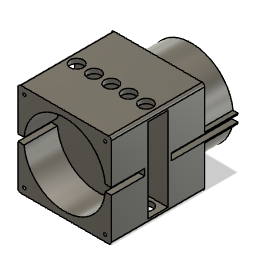
TWO MAG BODY 3x1 v13 (Autodesk Fusion 360 design; units mm, degrees)
Autodesk Fusion 360 part; units mm, degrees
sketch "Sketch3" plane through (0, 0, 0) normal (0, 0, 1) x (1, 0, 0)
  line L0 (44.45, 44.45) -> (-44.45, 44.45)
  line L1 (-44.45, 44.45) -> (-44.45, -44.45)
  line L2 (-44.45, -44.45) -> (44.45, -44.45)
  line L3 (44.45, -44.45) -> (44.45, 44.45)
  line L4 (44.45, 44.45) -> (-44.45, -44.45) construction
  line L5 (-44.45, 44.45) -> (44.45, -44.45) construction
  dimension "d6" = 88.9
  dimension "d7" = 88.9
  constraint perpendicular L0 L1
  constraint parallel L0 L2
  constraint parallel L1 L3
  constraint horizontal L0
  constraint coincident L4 origin
  constraint coincident L5 origin
  measures "d6" distance of L1.end L2.end
  measures "d7" distance of L0.end L1.end
extrude "Extrude2" add sketch "Sketch3" along normal mid plane 76.2
sketch "Sketch5" plane through (0, 0, 38.1) normal (0, 0, 1) x (1, 0, 0)
  line L0 (44.45, -44.45) -> (44.45, 44.45)
  line L1 (44.45, 44.45) -> (-44.45, 44.45)
  line L2 (-44.45, 44.45) -> (-44.45, -44.45)
  line L3 (-44.45, -44.45) -> (44.45, -44.45)
  circle A0 centre (0, 0) radius 38.735
  dimension "d14" = 77.47
  constraint coincident A0.centre origin
  measures "d14" diameter of A0
extrude "Extrude13" cut sketch "Sketch5" against normal blind 25.4 contours A0
sketch "Sketch10" plane through (44.45, 0, 0) normal (1, 0, 0) x (0, 0, -1)
  line L0 (38.1, 44.45) -> (-38.1, 44.45)
  line L1 (-38.1, 44.45) -> (-38.1, -44.45)
  line L2 (-38.1, -44.45) -> (38.1, -44.45)
  line L3 (38.1, -44.45) -> (38.1, 44.45)
  line L4 (9.525, 40.005) -> (-9.525, 40.005)
  line L5 (-9.525, 40.005) -> (-9.525, -40.005)
  line L6 (-9.525, -40.005) -> (9.525, -40.005)
  line L7 (9.525, -40.005) -> (9.525, 40.005)
  line L8 (9.525, 40.005) -> (-9.525, -40.005) construction
  line L9 (-9.525, 40.005) -> (9.525, -40.005) construction
  dimension "d42" = 80.01
  dimension "d43" = 19.05
  constraint perpendicular L4 L5
  constraint parallel L4 L6
  constraint parallel L5 L7
  constraint horizontal L4
  constraint coincident L8 origin
  constraint coincident L9 origin
  measures "d42" distance of L4.end L5.end
  measures "d43" distance of L5.end L6.end
extrude "Extrude9" cut sketch "Sketch10" against normal blind 88.9 contours L4 L5 L6 L7
sketch "Sketch6" plane through (0, 0, -38.1) normal (0, 0, -1) x (-1, 0, 0)
  line L0 (-44.45, 44.45) -> (-44.45, -44.45)
  line L1 (-44.45, -44.45) -> (44.45, -44.45)
  line L2 (44.45, -44.45) -> (44.45, 44.45)
  line L3 (44.45, 44.45) -> (-44.45, 44.45)
  circle A0 centre (0, 0) radius 38.735
  dimension "d17" = 77.47
  constraint coincident A0.centre origin
  measures "d17" diameter of A0
extrude "Extrude5" cut sketch "Sketch6" against normal blind 25.4 contours A0
sketch "Sketch7" plane through (44.45, 0, 0) normal (1, 0, 0) x (0, 0, -1)
  line L0 (38.1, 44.45) -> (-38.1, 44.45)
  line L1 (-38.1, 44.45) -> (-38.1, -44.45)
  line L2 (-38.1, -44.45) -> (38.1, -44.45)
  line L3 (38.1, -44.45) -> (38.1, 44.45)
  line L4 (-9.525, 40.005) -> (9.525, 40.005)
  line L5 (9.525, 40.005) -> (9.525, -40.005)
  line L6 (9.525, -40.005) -> (-9.525, -40.005)
  line L7 (-9.525, -40.005) -> (-9.525, 40.005)
  line L8 (-12.7, 3.175) -> (-12.7, -3.175)
  line L9 (-38.1, 3.175) -> (-38.1, -3.175)
  line L10 (12.7, -3.175) -> (12.7, 3.175)
  line L11 (38.1, -3.175) -> (38.1, 3.175)
  line L12 (12.7, 3.175) -> (38.1, 3.175)
  line L13 (38.1, -3.175) -> (12.7, -3.175)
  line L14 (-12.7, -3.175) -> (-38.1, -3.175)
  line L15 (-38.1, 3.175) -> (-12.7, 3.175)
  point P0 (-19.05, 0)
  constraint coincident L1 L9.start
  constraint coincident L1 L9.end
  constraint perpendicular L11 L12
  constraint perpendicular L10 L13
  constraint perpendicular L1 L14
  constraint perpendicular L8 L15
extrude "Extrude6" cut sketch "Sketch7" against normal blind 88.9 contours L3 L10 L11 L12 L13 | L1 L8 L9 L14 L15 | L4 L5 L6 L7
sketch "Sketch8" plane through (0, 0, 38.1) normal (0, 0, 1) x (1, 0, 0)
  line L0 (-44.45, -3.175) -> (-44.45, -44.45)
  line L1 (-44.45, -44.45) -> (44.45, -44.45)
  line L2 (44.45, -44.45) -> (44.45, -3.175)
  line L3 (-44.45, -44.45) -> (-44.45, -38.45) construction
  line L4 (-44.45, -38.45) -> (-38.45, -38.45) construction
  circle A0 centre (-38.45, -38.45) radius 1.4
  line L5 (0, 0) -> (0, -44.45) construction
  circle A1 centre (38.45, -38.45) radius 1.4
  circle A2 centre (38.45, 38.45) radius 1.4
  circle A3 centre (-38.45, 38.45) radius 1.4
  line L6 (44.45, -3.175) -> (38.6047, -3.175)
  arc A4 (-38.6047, -3.175) -> (38.6047, -3.175) centre (0, 0) ccw
  line L7 (-38.6047, -3.175) -> (-44.45, -3.175)
  dimension "d26" = 6
  dimension "d27" = 6
  dimension "d28" = 2.8
  dimension "d31" = 360
  constraint coincident L0.end L1.start
  constraint perpendicular L1 L3
  constraint perpendicular L3 L4
  constraint coincident L4.end A0.centre
  constraint midpoint L1 L5.end
  measures "d26" distance of L0.end L3.end
  measures "d27" distance of L3.end L4.end
  measures "d28" diameter of A0
extrude "Extrude7" cut sketch "Sketch8" against normal blind 7 contours A0 | A1 | A2 | A3
sketch "Sketch9" plane through (0, 0, -38.1) normal (0, 0, -1) x (-1, 0, 0)
  arc A0 (-38.6047, -3.175) -> (38.6047, -3.175) centre (0, 0) ccw
  line L0 (-44.45, -3.175) -> (-44.45, -44.45)
  line L1 (-44.45, -44.45) -> (44.45, -44.45)
  line L2 (44.45, -44.45) -> (44.45, -3.175)
  line L3 (-44.45, -44.45) -> (-44.45, -38.45) construction
  line L4 (-44.45, -38.45) -> (-38.45, -38.45) construction
  circle A1 centre (-38.45, -38.45) radius 1.4
  circle A2 centre (38.45, -38.45) radius 1.4
  circle A3 centre (38.45, 38.45) radius 1.4
  circle A4 centre (-38.45, 38.45) radius 1.4
  line L5 (44.45, -3.175) -> (38.6047, -3.175)
  line L6 (-38.6047, -3.175) -> (-44.45, -3.175)
  dimension "d34" = 6
  dimension "d35" = 6
  dimension "d36" = 2.8
  dimension "d38" = 360
  constraint coincident L0.end L1.start
  constraint perpendicular L1 L3
  constraint perpendicular L0 L4
  constraint coincident L4.end A1.centre
  measures "d34" distance of L0.end L3.end
  measures "d35" distance of L3.end L4.end
  measures "d36" diameter of A1
extrude "Extrude8" cut sketch "Sketch9" against normal blind 7 contours A1 | A2 | A3 | A4
fillet "Fillet1" radius 2.54 4 edges at (44.45, 44.45, 0) (-44.45, 44.45, 0) (44.45, -44.45, 0) (-44.45, -44.45, 0)
sketch "Sketch11" plane through (0, -44.45, 0) normal (0, -1, 0) x (1, 0, 0)
  line L0 (-41.91, 38.1) -> (-41.91, -38.1)
  line L1 (-41.91, -38.1) -> (41.91, -38.1)
  line L2 (41.91, -38.1) -> (41.91, 38.1)
  line L3 (41.91, 38.1) -> (-41.91, 38.1)
  circle A0 centre (0, 0) radius 6.35
  line L4 (0, 0) -> (41.91, 0) construction
  line L5 (0, 0) -> (-41.91, 0) construction
  line L6 (-6.35, 0) -> (-16.51, 0) construction
  circle A1 centre (-16.51, 0) radius 6.35
  line L7 (-22.86, 0) -> (-33.02, 0) construction
  circle A2 centre (-33.02, 0) radius 6.35
  circle A3 centre (16.51, 0) radius 6.35
  circle A4 centre (33.02, 0) radius 6.35
  dimension "d84" = 12.7
  dimension "d85" = 10.16
  dimension "d86" = 12.7
  dimension "d88" = 10.16
  dimension "d89" = 12.7
  dimension "d91" = 360
  constraint coincident A0.centre L4.start
  constraint midpoint L2 L4.end
  constraint midpoint L0 L5.end
  constraint coincident L5 L6.start
  constraint coincident A0 L6.start
  constraint parallel L5 L6
  constraint coincident L6.end A1.centre
  constraint coincident A1 L7.start
  constraint coincident L5 L7.start
  constraint parallel L5 L7
  constraint coincident L7.end A2.centre
  measures "d84" diameter of A0
  measures "d85" distance of L6.start L6.end
  measures "d86" diameter of A1
  measures "d88" distance of L7.start L7.end
  measures "d89" diameter of A2
extrude "Extrude14" cut sketch "Sketch11" against normal blind 88.9 contours A0 | A1 | A2 | A3 | A4
sketch "Sketch15" plane through (0, 0, -38.1) normal (0, 0, -1) x (-1, 0, 0)
  circle A0 centre (-38.45, 38.45) radius 1.4
  circle A1 centre (38.45, 38.45) radius 1.4
  arc A2 (44.45, 41.91) -> (41.91, 44.45) centre (41.91, 41.91) ccw
  line L0 (41.91, 44.45) -> (-41.91, 44.45)
  arc A3 (-41.91, 44.45) -> (-44.45, 41.91) centre (-41.91, 41.91) ccw
  line L1 (-44.45, 41.91) -> (-44.45, 3.175)
  line L2 (-44.45, 3.175) -> (-38.6047, 3.175)
  arc A4 (38.6047, 3.175) -> (-38.6047, 3.175) centre (0, 0) ccw
  line L3 (38.6047, 3.175) -> (44.45, 3.175)
  line L4 (44.45, 3.175) -> (44.45, 41.91)
  line L5 (-38.6047, 3.175) -> (-44.45, 3.175)
  line L6 (-44.45, 3.175) -> (-44.45, 4.375)
  arc A5 (39.6946, 4.375) -> (-39.6946, 4.375) centre (0, 0) ccw
  arc A6 (38.6047, 3.175) -> (-38.6047, 3.175) centre (0, 0) ccw
  line L7 (-44.45, 4.375) -> (-39.6946, 4.375)
  line L8 (38.6047, 3.175) -> (44.45, 3.175)
  line L9 (44.45, 3.175) -> (44.45, 4.375)
  line L10 (44.45, 4.375) -> (39.6946, 4.375)
  arc A7 (-39.6946, -4.375) -> (39.6946, -4.375) centre (0, 0) ccw
  arc A8 (-38.6047, -3.175) -> (38.6047, -3.175) centre (0, 0) ccw
  line L11 (38.6047, -3.175) -> (44.45, -3.175)
  line L12 (44.45, -4.375) -> (39.6946, -4.375)
  line L13 (-38.6047, -3.175) -> (-44.45, -3.175)
  line L14 (-44.45, -4.375) -> (-39.6946, -4.375)
  line L15 (-44.45, -3.175) -> (-44.45, -4.375)
  line L16 (44.45, -3.175) -> (44.45, -4.375)
  dimension "d95" = 1.2
  dimension "d96" = 1.2
  dimension "d98" = 360
  constraint concentric A4 A6
  constraint concentric A5 A6
  constraint coincident L2.end A4.end
  constraint coincident L1.end L2.start
  constraint perpendicular L5 L6
  constraint perpendicular L6 L7
  constraint coincident A4.start L3.start
  constraint coincident L3.end L4.start
  constraint perpendicular L8 L9
  constraint perpendicular L9 L10
  measures "d95" distance of L1.end L6.end
  measures "d96" distance of L3.end L9.end
extrude "Extrude15" add sketch "Sketch15" along normal blind 38.1 contours L1 L2 A4 L3 L4 L5 L6 A5 A6 L7 L8 L9 L10 | A7 A8 L11 L12 L13 L14 L15 L16
extrude "Extrude16" add 2 faces at (-41.8839, 20.6364, -38.1) (-41.8839, -20.6364, -38.1) along direction (0, 0, -1) blind 6.35
extrude "Extrude17" add 2 faces at (-41.6249, 19.8152, 38.1) (-41.6249, -19.8152, 38.1) along direction (0, 0, 1) blind 6.35
